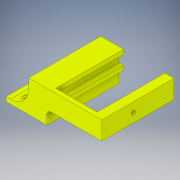
# Autodesk Inventor part: batterybracket4
Saved by Autodesk Inventor 2017 (Build 210142000, 142)
## iProperties
Created: 2017-08-12
Part Number: batterybracket4
Material: Generic
Document SubType Name: Modeling
Designer: Kai
Density: 1 g/cm^3
Appearance: Default
Author: Kai
Autodesk Inventor part; units mm, degrees
ref_plane "YZ Plane" through (0, 0, 0) normal (1, 0, 0) x (0, 1, 0)
ref_plane "XZ Plane" through (0, 0, 0) normal (0, 1, 0) x (-1, 0, 0)
ref_plane "XY Plane" through (0, 0, 0) normal (0, 0, 1) x (1, 0, 0)
sketch "Sketch1" plane through (0, 0, 0) normal (0, 0, 1) x (1, 0, 0)
  line L0 (77.3388, 19.558) -> (77.3388, -6.35)
  line L1 (-6.35, -6.35) -> (-6.35, 19.558)
  line L2 (6.35, 19.558) -> (6.35, 13.208)
  line L3 (0, 13.208) -> (0, 0)
  line L4 (6.35, 0) -> (6.35, -6.35)
  line L5 (69.85, 13.208) -> (69.85, 0)
  line L6 (64.6388, 19.558) -> (64.6388, 13.208)
  line L7 (64.6388, 0) -> (64.6388, -6.35)
  line L8 (-6.35, 19.558) -> (6.35, 19.558)
  line L9 (64.6388, 19.558) -> (77.3388, 19.558)
  line L10 (69.85, 13.208) -> (64.6388, 13.208)
  line L11 (6.35, 13.208) -> (0, 13.208)
  line L12 (0, 0) -> (6.35, 0)
  line L13 (64.6388, 0) -> (69.85, 0)
  line L14 (77.3388, -6.35) -> (64.6388, -6.35)
  line L15 (6.35, -6.35) -> (-6.35, -6.35)
  dimension "d0" = 69.85
  dimension "d1" = 13.208
  dimension "d3" = 12.7
  dimension "d4" = 12.7
  constraints: 32 end point, 9 parallel, 8 perpendicular, 4 point on line, 2 horizontal, 1 vertical
  measures "d0" distance of L3.start L5.start
  measures "d1" distance of L5.start L5.end
  measures "d3" distance between parallel lines of L1 L2
  measures "d4" distance between parallel lines of L0 L6
extrude "Extrusion1" add sketch "Sketch1" along normal blind 114.3
sketch "Sketch2" plane through (0, 0, 0) normal (0, 0, -1) x (-1, 0, 0)
  line L0 (-77.3388, 19.558) -> (-64.6388, 19.558) projected
  line L1 (6.35, -6.35) -> (-77.3388, -6.35)
  line L2 (-77.3388, -6.35) -> (-77.3388, 19.558)
  line L3 (-77.3388, 19.558) -> (6.35, 19.558)
  line L4 (6.35, 19.558) -> (25.4, 19.558)
  line L5 (25.4, 19.558) -> (25.4, -6.35)
  line L6 (25.4, -6.35) -> (6.35, -6.35)
  point P0 (0, 0)
  dimension "d46" = 19.05
  constraints: 12 end point, 3 perpendicular, 2 horizontal, 1 parallel
  measures "d46" distance of L3.end L4.end
extrude "Extrusion2" add sketch "Sketch2" along normal blind 6.35
sketch "Sketch3" plane through (0, 0, 114.3) normal (0, 0, 1) x (1, 0, 0)
  line L0 (-25.4, 19.558) -> (77.3388, 19.558) projected
  line L1 (0, 19.558) -> (-6.35, 19.558)
  line L2 (-57.15, -19.05) -> (-57.15, -25.4)
  line L3 (-57.15, -25.4) -> (0, -25.4)
  line L4 (0, -25.4) -> (0, 19.558)
  line L5 (-6.35, 19.558) -> (-6.35, 6.35)
  line L6 (6.35, 0) -> (0, 0) projected
  line L7 (-6.35, 19.558) -> (-25.4, 19.558)
  line L8 (-25.4, 19.558) -> (-25.4, 6.35)
  line L9 (-50.8, -19.05) -> (-57.15, -19.05)
  arc A0 (-50.8, -19.05) -> (-25.4, 6.35) centre (-50.8, 6.35) ccw
  point P0 (-6.35, -6.35)
  point P1 (-6.35, -19.05)
  dimension "d9" = 57.15
  dimension "d11" = 12.7
  dimension "d40" = 25.4
  dimension "d47" = 25.4
  constraints: 16 end point, 3 point on line, 2 horizontal, 2 parallel, 2 perpendicular, 2 point on circle, 2 tangent, 1 centre point, 1 vertical
  measures "d9" distance of L3.end L2.end
  measures "d11" distance of point (-6.35, -6.35) point (-6.35, -19.05)
  measures "d40" distance from line of L6 L3.end
  measures "d47" radius of A0
extrude "Extrusion3" add sketch "Sketch3" against normal up to surface (120.65 mm away)
sketch "Sketch4" plane through (-57.15, -25.4, 114.3) normal (0, -1, 0) x (1, 0, 0)
  line L0 (6.35, 0) -> (31.75, 0) construction
  line L1 (19.05, 0) -> (17.3485, -120.65) construction
  line L2 (6.35, -120.65) -> (6.35, -120.65) construction
  circle A0 centre (17.5276, -107.95) radius 3.1
  circle A1 centre (17.8858, -82.5525) radius 3.1
  circle A2 centre (18.244, -57.1551) radius 3.1
  circle A3 centre (18.6021, -31.7576) radius 3.1
  point P0 (57.15, -114.3)
  point P1 (28.347, -120.65)
  dimension "d16" = 6.2
  dimension "d17" = 12.7
  dimension "d20" = 25.4
  constraints: 4 centre point, 2 end point, 1 midpoint, 1 point on line, 9 other
  measures "d16" diameter of A0
  measures "d20" distance of A0.centre A1.centre
extrude "Extrusion4" cut sketch "Sketch4" against normal blind 101.6
fillet "Fillet1" radius 6.35 1 edges at (0, -6.35, 53.975)
sketch "Sketch6" plane through (0, 0, 114.3) normal (0, 0, 1) x (1, 0, 0)
  line L0 (-57.15, -19.05) -> (-57.15, -25.4) projected
  line L1 (77.3388, 19.558) -> (64.6388, 19.558) projected
  line L2 (-57.15, -25.4) -> (77.3388, -25.4)
  line L3 (77.3388, -25.4) -> (77.3388, 19.558)
  line L4 (77.3388, 19.558) -> (-57.15, 19.558)
  line L5 (-57.15, 19.558) -> (-57.15, -25.4)
  point P0 (0, 0)
  constraints: 8 end point, 2 parallel, 1 horizontal, 1 perpendicular
extrude "Extrusion6" cut sketch "Sketch6" against normal blind 19.05
sketch "Sketch7" plane through (77.3388, -6.35, -6.35) normal (1, 0, 0) x (0, 0, -1)
  circle A0 centre (-44.45, 12.7) radius 2.85
  line L0 (0, 25.908) -> (0, 0) projected
  line L1 (0, 0) -> (-101.6, 0) projected
  point P0 (-6.35, 6.35)
  dimension "d41" = 5.7
  dimension "d42" = 44.45
  dimension "d43" = 12.7
  constraints: 1 centre point
  measures "d41" diameter of A0
  measures "d42" distance from line of L0 A0.centre
  measures "d43" distance from line of L1 A0.centre
extrude "Extrusion7" cut sketch "Sketch7" against normal blind 25.4
sketch "Sketch8" plane through (-57.15, -19.05, -6.35) normal (0, 1, 0) x (1, 0, 0)
  line L0 (6.35, 0) -> (0, 0) construction
  line L1 (0, 0) -> (0, -14.734) construction
  line L2 (0, -101.6) -> (0, 0) construction
  circle A0 centre (17.5276, -12.7) radius 3.1 projected
  circle A1 centre (17.5276, -12.7) radius 6
  circle A2 centre (17.8858, -38.0975) radius 3.1 construction
  line L3 (17.5276, -12.7) -> (17.8858, -38.0975) construction
  circle A3 centre (17.8858, -38.0975) radius 6
  circle A4 centre (18.244, -63.4949) radius 6
  circle A5 centre (18.6021, -88.8924) radius 6
  point P0 (57.15, -6.35)
  dimension "d48" = 12
  dimension "d51" = 25.4
  constraints: 4 centre point, 4 end point, 1 coincident, 1 point on line, 7 other
  measures "d48" diameter of A1
  measures "d51" distance of A1.centre A3.centre
extrude "Extrusion8" cut sketch "Sketch8" along normal blind 25.4
mirror "Mirror1" about plane through (10.0944, -2.921, 95.25) normal (0, 0, 1) remove original yes
body "Solid1"
